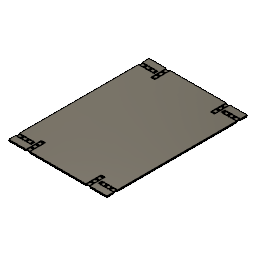
E-Reader Case v2 (Autodesk Fusion 360 design; units mm, degrees)
Autodesk Fusion 360 part; units mm, degrees
sketch "Sketch1" plane through (0, 0, 0) normal (0, 1, 0) x (1, 0, 0)
  line L0 (0, 0) -> (140, 0)
  line L1 (140, 0) -> (140, -200)
  line L2 (140, -200) -> (0, -200)
  line L3 (0, -200) -> (0, 0)
  dimension "d1" = 140
  dimension "d2" = 200
  constraint horizontal L0
  constraint vertical L1
  constraint horizontal L2
  constraint vertical L3
  constraint coincident L0.start L3.end
  measures "d1" distance of L0.start L0.end
  measures "d2" distance of L0.start L2.end
extrude "Extrude1" add sketch "Sketch1" along normal blind 2
sketch "Sketch2" plane through (0, 2, 0) normal (0, 1, 0) x (-1, 0, 0)
  line L0 (0, 200) -> (-140, 200)
  line L1 (-140, 200) -> (-140, 0)
  line L2 (-140, 0) -> (0, 0)
  line L3 (0, 0) -> (0, 200)
  line L4 (0, 0) -> (-30, 0)
  line L5 (-30, 0) -> (-30, 15)
  line L6 (-30, 15) -> (0, 15)
  line L7 (0, 15) -> (0, 0)
  line L8 (-140, 0) -> (-110, 0)
  line L9 (-110, 0) -> (-110, 15)
  line L10 (-110, 15) -> (-140, 15)
  line L11 (-140, 15) -> (-140, 0)
  line L12 (0, 200) -> (-30, 200)
  line L13 (-30, 200) -> (-30, 185)
  line L14 (-30, 185) -> (0, 185)
  line L15 (0, 185) -> (0, 200)
  line L16 (-140, 200) -> (-110, 200)
  line L17 (-110, 200) -> (-110, 185)
  line L18 (-110, 185) -> (-140, 185)
  line L19 (-140, 185) -> (-140, 200)
  line L20 (-110, 200) -> (-113, 200)
  line L21 (-140, 185) -> (-139, 185)
  line L22 (-110, 200) -> (-110, 199)
  line L23 (-120.831, 200) -> (-110, 200)
  line L24 (-110, 200) -> (-110, 199)
  line L25 (-30, 200) -> (-25, 200)
  line L26 (-25, 200) -> (-25, 199)
  line L27 (-25, 199) -> (-30, 199)
  line L28 (-30, 199) -> (-30, 200)
  line L29 (0, 185) -> (-1, 185)
  line L30 (-1, 185) -> (-1, 190)
  line L31 (-1, 190) -> (0, 190)
  line L32 (0, 190) -> (0, 185)
  line L33 (-140, 15) -> (-139, 15)
  line L34 (-139, 15) -> (-139, 10)
  line L35 (-139, 10) -> (-140, 10)
  line L36 (-140, 10) -> (-140, 15)
  line L37 (-110, 0) -> (-115, 0)
  line L38 (-115, 0) -> (-115, 1)
  line L39 (-115, 1) -> (-110, 1)
  line L40 (-110, 1) -> (-110, 0)
  line L41 (-30, 0) -> (-25, 0)
  line L42 (-25, 0) -> (-25, 1)
  line L43 (-25, 1) -> (-30, 1)
  line L44 (-30, 1) -> (-30, 0)
  line L45 (0, 15) -> (-1, 15)
  line L46 (-1, 15) -> (-1, 10)
  line L47 (-1, 10) -> (0, 10)
  line L48 (0, 10) -> (0, 15)
  line L49 (-140, 185) -> (-139, 185)
  line L50 (-139, 185) -> (-139, 190)
  line L51 (-139, 190) -> (-140, 190)
  line L52 (-140, 190) -> (-140, 185)
  line L53 (-110, 200) -> (-115, 200)
  line L54 (-115, 200) -> (-115, 199)
  line L55 (-115, 199) -> (-110, 199)
  line L56 (-110, 199) -> (-110, 200)
  dimension "d5" = 30
  dimension "d6" = 15
  dimension "d7" = 30
  dimension "d8" = 15
  dimension "d9" = 30
  dimension "d10" = 15
  dimension "d11" = 30
  dimension "d12" = 15
  dimension "d13" = 3
  dimension "d18" = 1
  dimension "d19" = 1
  dimension "d20" = 5
  dimension "d21" = 1
  dimension "d22" = 1
  dimension "d23" = 5
  dimension "d24" = 1
  dimension "d25" = 5
  dimension "d26" = 5
  dimension "d27" = 1
  dimension "d28" = 5
  dimension "d29" = 1
  dimension "d30" = 1
  dimension "d31" = 5
  dimension "d34" = 1
  dimension "d35" = 5
  dimension "d36" = 5
  dimension "d37" = 1
  constraint horizontal L4
  constraint vertical L5
  constraint horizontal L6
  constraint vertical L7
  constraint coincident L2.end L3.start
  constraint horizontal L8
  constraint vertical L9
  constraint horizontal L10
  constraint vertical L11
  constraint coincident L1.end L2.start
  constraint horizontal L12
  constraint vertical L13
  constraint horizontal L14
  constraint vertical L15
  constraint coincident L0.start L3.end
  constraint horizontal L16
  constraint vertical L17
  constraint horizontal L18
  constraint vertical L19
  constraint coincident L0.end L1.start
  constraint perpendicular L17 L20
  constraint horizontal L21
  constraint perpendicular L20 L22
  constraint horizontal L23
  constraint vertical L24
  constraint coincident L16 L23.start
  constraint horizontal L25
  constraint vertical L26
  constraint horizontal L27
  constraint vertical L28
  constraint horizontal L29
  constraint vertical L30
  constraint horizontal L31
  constraint vertical L32
  constraint horizontal L33
  constraint vertical L34
  constraint horizontal L35
  constraint vertical L36
  constraint horizontal L37
  constraint vertical L38
  constraint horizontal L39
  constraint vertical L40
  constraint horizontal L41
  constraint vertical L42
  constraint horizontal L43
  constraint vertical L44
  constraint horizontal L45
  constraint vertical L46
  constraint horizontal L47
  constraint vertical L48
  constraint horizontal L49
  constraint vertical L50
  constraint horizontal L51
  constraint vertical L52
  constraint horizontal L53
  constraint vertical L54
  constraint horizontal L55
  constraint vertical L56
  measures "d5" distance of L2.end L4.end
  measures "d6" distance of L2.end L6.end
  measures "d7" distance of L1.end L8.end
  measures "d8" distance of L1.end L10.end
  measures "d9" distance of L0.start L12.end
  measures "d10" distance of L0.start L14.end
  measures "d11" distance of L0.end L16.end
  measures "d12" distance of L0.end L18.end
  measures "d13" distance of L16.end L20.end
  measures "d18" distance of L18.end L21.end
  measures "d19" distance of L16.end L22.end
  measures "d20" distance of L12.end L25.end
  measures "d21" distance of L12.end L27.end
  measures "d22" distance of L14.end L29.end
  measures "d23" distance of L14.end L31.end
  measures "d24" distance of L10.end L33.end
  measures "d25" distance of L10.end L35.end
  measures "d26" distance of L8.end L37.end
  measures "d27" distance of L8.end L39.end
  measures "d28" distance of L4.end L41.end
  measures "d29" distance of L4.end L43.end
  measures "d30" distance of L6.end L45.end
  measures "d31" distance of L6.end L47.end
  measures "d34" distance of L18.end L21.end
  measures "d35" distance of L18.end L51.end
  measures "d36" distance of L16.end L53.end
  measures "d37" distance of L16.end L22.end
extrude "Extrude2" cut sketch "Sketch2" against normal blind 2 contours L0 L12 L13 L25 L26 L27 L28 | L3 L14 L15 L29 L30 L31 L32 | L0 L16 L17 L20 L22 L23 L24 L53 L54 L55 L56 | L3 L6 L7 L45 L46 L47 L48 | L1 L18 L19 L21 L49 L50 L51 L52 | L2 L4 L5 L41 L42 L43 L44 | L1 L10 L11 L33 L34 L35 L36 | L2 L8 L9 L37 L38 L39 L40
sketch "Sketch3" plane through (0, 2, 0) normal (0, 1, 0) x (-1, 0, 0)
  line L0 (-110, 1) -> (-110, 0)
  line L1 (-110, 0) -> (-30, 0)
  line L2 (-30, 0) -> (-30, 1)
  line L3 (-30, 1) -> (-25, 1)
  line L4 (-25, 0) -> (0, 0)
  line L5 (0, 0) -> (0, 10)
  line L6 (0, 10) -> (-1, 10)
  line L7 (-1, 10) -> (-1, 15)
  line L8 (-1, 15) -> (0, 15)
  line L9 (0, 15) -> (0, 185)
  line L10 (0, 185) -> (-1, 185)
  line L11 (-1, 185) -> (-1, 190)
  line L12 (-1, 190) -> (0, 190)
  line L13 (0, 190) -> (0, 200)
  line L14 (0, 200) -> (-25, 200)
  line L15 (-25, 200) -> (-25, 199)
  line L16 (-25, 199) -> (-30, 199)
  line L17 (-30, 199) -> (-30, 200)
  line L18 (-30, 200) -> (-110, 200)
  line L19 (-110, 200) -> (-110, 199)
  line L20 (-110, 199) -> (-115, 199)
  line L21 (-115, 199) -> (-115, 200)
  line L22 (-115, 200) -> (-140, 200)
  line L23 (-140, 200) -> (-140, 190)
  line L24 (-140, 190) -> (-139, 190)
  line L25 (-139, 190) -> (-139, 185)
  line L26 (-139, 185) -> (-140, 185)
  line L27 (-140, 185) -> (-140, 15)
  line L28 (-140, 15) -> (-139, 15)
  line L29 (-139, 15) -> (-139, 10)
  line L30 (-139, 10) -> (-140, 10)
  line L31 (-140, 10) -> (-140, 0)
  line L32 (-140, 0) -> (-115, 0)
  line L33 (-115, 1) -> (-110, 1)
  line L34 (-110, 199) -> (-115, 199)
  line L35 (-115, 199) -> (-115, 194)
  line L36 (-115, 194) -> (-110, 194)
  line L37 (-110, 194) -> (-110, 199)
  line L38 (-110, 194) -> (-115, 194)
  line L39 (-115, 194) -> (-115, 192)
  line L40 (-115, 192) -> (-110, 192)
  line L41 (-110, 192) -> (-110, 194)
  line L42 (-115, 192) -> (-110, 192)
  line L43 (-110, 192) -> (-110, 187)
  line L44 (-110, 187) -> (-115, 187)
  line L45 (-115, 187) -> (-115, 192)
  line L46 (-110, 187) -> (-115, 187)
  line L47 (-115, 187) -> (-115, 185)
  line L48 (-115, 185) -> (-110, 185)
  line L49 (-110, 185) -> (-110, 187)
  line L50 (-139, 185) -> (-134, 185)
  line L51 (-134, 185) -> (-134, 190)
  line L52 (-134, 190) -> (-139, 190)
  line L53 (-139, 190) -> (-139, 185)
  line L54 (-134, 190) -> (-132, 190)
  line L55 (-132, 190) -> (-132, 185)
  line L56 (-132, 185) -> (-134, 185)
  line L57 (-134, 185) -> (-134, 190)
  line L58 (-132, 185) -> (-127, 185)
  line L59 (-127, 185) -> (-127, 190)
  line L60 (-127, 190) -> (-132, 190)
  line L61 (-132, 190) -> (-132, 185)
  line L62 (-127, 190) -> (-125, 190)
  line L63 (-125, 190) -> (-125, 185)
  line L64 (-125, 185) -> (-127, 185)
  line L65 (-127, 185) -> (-127, 190)
  line L66 (-25, 199) -> (-30, 199)
  line L67 (-30, 199) -> (-30, 194)
  line L68 (-30, 194) -> (-25, 194)
  line L69 (-25, 194) -> (-25, 199)
  line L70 (-30, 194) -> (-25, 194)
  line L71 (-25, 194) -> (-25, 192)
  line L72 (-25, 192) -> (-30, 192)
  line L73 (-30, 192) -> (-30, 194)
  line L74 (-25, 192) -> (-30, 192)
  line L75 (-30, 192) -> (-30, 187)
  line L76 (-30, 187) -> (-25, 187)
  line L77 (-25, 187) -> (-25, 192)
  line L78 (-25, 187) -> (-30, 187)
  line L79 (-30, 187) -> (-30, 185)
  line L80 (-30, 185) -> (-25, 185)
  line L81 (-25, 185) -> (-25, 187)
  line L82 (-30, 185) -> (-25, 185)
  line L83 (-25, 185) -> (-25, 180)
  line L84 (-25, 180) -> (-30, 180)
  line L85 (-30, 180) -> (-30, 185)
  line L86 (-110, 185) -> (-115, 185)
  line L87 (-115, 185) -> (-115, 180)
  line L88 (-115, 180) -> (-110, 180)
  line L89 (-110, 180) -> (-110, 185)
  line L90 (-125, 185) -> (-120, 185)
  line L91 (-120, 185) -> (-120, 190)
  line L92 (-120, 190) -> (-125, 190)
  line L93 (-125, 190) -> (-125, 185)
  line L94 (-1, 185) -> (-6, 185)
  line L95 (-6, 185) -> (-6, 190)
  line L96 (-6, 190) -> (-1, 190)
  line L97 (-1, 190) -> (-1, 185)
  line L98 (-6, 190) -> (-8, 190)
  line L99 (-8, 190) -> (-8, 185)
  line L100 (-8, 185) -> (-6, 185)
  line L101 (-6, 185) -> (-6, 190)
  line L102 (-8, 185) -> (-13, 185)
  line L103 (-13, 185) -> (-13, 190)
  line L104 (-13, 190) -> (-8, 190)
  line L105 (-8, 190) -> (-8, 185)
  line L106 (-13, 190) -> (-15, 190)
  line L107 (-15, 190) -> (-15, 185)
  line L108 (-15, 185) -> (-13, 185)
  line L109 (-13, 185) -> (-13, 190)
  line L110 (-15, 185) -> (-20, 185)
  line L111 (-20, 185) -> (-20, 190)
  line L112 (-20, 190) -> (-15, 190)
  line L113 (-15, 190) -> (-15, 185)
  line L114 (-120, 15) -> (-125, 15)
  line L115 (-125, 10) -> (-120, 10)
  line L116 (-132, 15) -> (-132, 10)
  line L117 (-125, 15) -> (-125, 10)
  line L118 (-125, 10) -> (-127, 10)
  line L119 (-127, 10) -> (-127, 15)
  line L120 (-134, 15) -> (-132, 15)
  line L121 (-139, 10) -> (-134, 10)
  line L122 (-127, 15) -> (-132, 15)
  line L123 (-127, 10) -> (-127, 15)
  line L124 (-134, 10) -> (-134, 15)
  line L125 (-127, 15) -> (-125, 15)
  line L126 (-125, 15) -> (-125, 10)
  line L127 (-134, 15) -> (-139, 15)
  line L128 (-132, 10) -> (-134, 10)
  line L129 (-132, 10) -> (-127, 10)
  line L130 (-139, 15) -> (-139, 10)
  line L131 (-134, 10) -> (-134, 15)
  line L132 (-132, 15) -> (-132, 10)
  line L133 (-139, 15) -> (-139, 10)
  line L134 (-1, 15) -> (-6, 15)
  line L135 (-6, 10) -> (-1, 10)
  line L136 (-13, 15) -> (-13, 10)
  line L137 (-6, 15) -> (-6, 10)
  line L138 (-6, 10) -> (-8, 10)
  line L139 (-8, 10) -> (-8, 15)
  line L140 (-15, 15) -> (-13, 15)
  line L141 (-20, 10) -> (-15, 10)
  line L142 (-8, 15) -> (-13, 15)
  line L143 (-8, 10) -> (-8, 15)
  line L144 (-15, 10) -> (-15, 15)
  line L145 (-8, 15) -> (-6, 15)
  line L146 (-6, 15) -> (-6, 10)
  line L147 (-1, 12) -> (-1, 10)
  line L148 (-15, 15) -> (-20, 15)
  line L149 (-13, 10) -> (-15, 10)
  line L150 (-13, 10) -> (-8, 10)
  line L151 (-15, 10) -> (-15, 15)
  line L152 (-13, 15) -> (-13, 10)
  line L153 (-1, 10) -> (-1, 15)
  line L154 (-120, 190) -> (-118, 190)
  line L155 (-118, 190) -> (-118, 185)
  line L156 (-118, 185) -> (-120, 185)
  line L157 (-120, 185) -> (-120, 190)
  line L158 (-110, 180) -> (-115, 180)
  line L159 (-115, 180) -> (-115, 178)
  line L160 (-115, 178) -> (-110, 178)
  line L161 (-110, 178) -> (-110, 180)
  line L162 (-20, 185) -> (-22, 185)
  line L163 (-22, 185) -> (-22, 190)
  line L164 (-22, 190) -> (-20, 190)
  line L165 (-20, 190) -> (-20, 185)
  line L166 (-25, 180) -> (-30, 180)
  line L167 (-30, 180) -> (-30, 178)
  line L168 (-30, 178) -> (-25, 178)
  line L169 (-25, 178) -> (-25, 180)
  line L170 (-20, 15) -> (-20, 10)
  line L171 (-20, 15) -> (-22, 15)
  line L172 (-22, 15) -> (-22, 10)
  line L173 (-22, 10) -> (-20, 10)
  line L174 (-20, 10) -> (-20, 15)
  line L175 (-120, 15) -> (-118, 15)
  line L176 (-118, 15) -> (-118, 10)
  line L177 (-118, 10) -> (-120, 10)
  line L178 (-120, 10) -> (-120, 15)
  line L179 (-115, 8) -> (-115, 13)
  line L180 (-110, 13) -> (-110, 15)
  line L181 (-115, 13) -> (-110, 13)
  line L182 (-110, 20) -> (-115, 20)
  line L183 (-115, 6) -> (-115, 1)
  line L184 (-110, 6) -> (-115, 6)
  line L185 (-110, 8) -> (-115, 8)
  line L186 (-115, 15) -> (-115, 13)
  line L187 (-110, 8) -> (-115, 8)
  line L188 (-110, 20) -> (-115, 20)
  line L189 (-110, 15) -> (-110, 20)
  line L190 (-115, 13) -> (-110, 13)
  line L191 (-110, 13) -> (-110, 8)
  line L192 (-110, 1) -> (-115, 1)
  line L193 (-115, 8) -> (-115, 6)
  line L194 (-115, 20) -> (-115, 15)
  line L195 (-115, 1) -> (-110, 1)
  line L196 (-115, 6) -> (-110, 6)
  line L197 (-115, 15) -> (-110, 15)
  line L198 (-110, 6) -> (-110, 8)
  line L199 (-110, 15) -> (-115, 15)
  line L200 (-110, 1) -> (-110, 6)
  line L201 (-30, 8) -> (-30, 13)
  line L202 (-25, 13) -> (-25, 15)
  line L203 (-30, 13) -> (-25, 13)
  line L204 (-25, 20) -> (-30, 20)
  line L205 (-30, 6) -> (-30, 1)
  line L206 (-25, 6) -> (-30, 6)
  line L207 (-25, 8) -> (-30, 8)
  line L208 (-30, 15) -> (-30, 13)
  line L209 (-25, 8) -> (-30, 8)
  line L210 (-25, 20) -> (-30, 20)
  line L211 (-25, 15) -> (-25, 20)
  line L212 (-30, 13) -> (-25, 13)
  line L213 (-25, 13) -> (-25, 8)
  line L214 (-25, 1) -> (-30, 1)
  line L215 (-30, 8) -> (-30, 6)
  line L216 (-30, 20) -> (-30, 15)
  line L217 (-30, 1) -> (-25, 1)
  line L218 (-30, 6) -> (-25, 6)
  line L219 (-30, 15) -> (-25, 15)
  line L220 (-25, 6) -> (-25, 8)
  line L221 (-25, 15) -> (-30, 15)
  line L222 (-25, 1) -> (-25, 6)
  line L223 (-25, 20) -> (-30, 20)
  line L224 (-30, 20) -> (-30, 22)
  line L225 (-30, 22) -> (-25, 22)
  line L226 (-25, 22) -> (-25, 20)
  line L227 (-110, 20) -> (-115, 20)
  line L228 (-115, 20) -> (-115, 22)
  line L229 (-115, 22) -> (-110, 22)
  line L230 (-110, 22) -> (-110, 20)
  point P0 (-1, 10)
  point P1 (-1, 12)
  dimension "d38" = 5
  dimension "d39" = 5
  dimension "d40" = 5
  dimension "d41" = 2
  dimension "d42" = 5
  dimension "d43" = 5
  dimension "d44" = 5
  dimension "d45" = 2
  dimension "d46" = 5
  dimension "d47" = 5
  dimension "d48" = 2
  dimension "d49" = 5
  dimension "d50" = 5
  dimension "d51" = 5
  dimension "d52" = 2
  dimension "d53" = 5
  dimension "d54" = 5
  dimension "d55" = 5
  dimension "d56" = 5
  dimension "d57" = 2
  dimension "d58" = 5
  dimension "d59" = 5
  dimension "d60" = 5
  dimension "d61" = 2
  dimension "d62" = 5
  dimension "d63" = 5
  dimension "d64" = 5
  dimension "d65" = 5
  dimension "d66" = 5
  dimension "d67" = 5
  dimension "d68" = 5
  dimension "d69" = 5
  dimension "d70" = 2
  dimension "d71" = 5
  dimension "d72" = 5
  dimension "d73" = 5
  dimension "d74" = 2
  dimension "d75" = 5
  dimension "d76" = 5
  dimension "d77" = 5
  dimension "d78" = 5
  dimension "d79" = 5
  dimension "d80" = 2
  dimension "d81" = 5
  dimension "d82" = 5
  dimension "d83" = 5
  dimension "d84" = 2
  dimension "d85" = 5
  dimension "d86" = 5
  dimension "d87" = 5
  dimension "d88" = 5
  dimension "d90" = 2
  dimension "d91" = 5
  dimension "d92" = 5
  dimension "d93" = 5
  dimension "d94" = 2
  dimension "d95" = 5
  dimension "d96" = 5
  dimension "d97" = 5
  dimension "d126" = 2
  dimension "d127" = 5
  dimension "d128" = 2
  dimension "d129" = 2
  dimension "d130" = 5
  dimension "d131" = 2
  dimension "d132" = 2
  dimension "d133" = 2
  dimension "d134" = 5
  dimension "d135" = 5
  dimension "d136" = 5
  dimension "d137" = 2
  dimension "d138" = 5
  dimension "d139" = 5
  dimension "d140" = 5
  dimension "d141" = 2
  dimension "d142" = 5
  dimension "d143" = 5
  dimension "d144" = 5
  dimension "d145" = 5
  dimension "d146" = 5
  dimension "d147" = 5
  dimension "d148" = 2
  dimension "d149" = 5
  dimension "d150" = 5
  dimension "d151" = 5
  dimension "d152" = 2
  dimension "d153" = 5
  dimension "d154" = 5
  dimension "d155" = 5
  dimension "d156" = 2
  dimension "d157" = 2
  constraint horizontal L34
  constraint vertical L35
  constraint horizontal L36
  constraint vertical L37
  constraint coincident L19.end L20.start
  constraint horizontal L38
  constraint vertical L39
  constraint horizontal L40
  constraint vertical L41
  constraint horizontal L42
  constraint vertical L43
  constraint horizontal L44
  constraint vertical L45
  constraint horizontal L46
  constraint vertical L47
  constraint horizontal L48
  constraint vertical L49
  constraint horizontal L50
  constraint vertical L51
  constraint horizontal L52
  constraint vertical L53
  constraint coincident L25.end L26.start
  constraint horizontal L54
  constraint vertical L55
  constraint horizontal L56
  constraint vertical L57
  constraint horizontal L58
  constraint vertical L59
  constraint horizontal L60
  constraint vertical L61
  constraint horizontal L62
  constraint vertical L63
  constraint horizontal L64
  constraint vertical L65
  constraint horizontal L66
  constraint vertical L67
  constraint horizontal L68
  constraint vertical L69
  constraint coincident L15.end L16.start
  constraint horizontal L70
  constraint vertical L71
  constraint horizontal L72
  constraint vertical L73
  constraint horizontal L74
  constraint vertical L75
  constraint horizontal L76
  constraint vertical L77
  constraint horizontal L78
  constraint vertical L79
  constraint horizontal L80
  constraint vertical L81
  constraint horizontal L82
  constraint vertical L83
  constraint horizontal L84
  constraint vertical L85
  constraint horizontal L86
  constraint vertical L87
  constraint horizontal L88
  constraint vertical L89
  constraint horizontal L90
  constraint vertical L91
  constraint horizontal L92
  constraint vertical L93
  constraint horizontal L94
  constraint vertical L95
  constraint horizontal L96
  constraint vertical L97
  constraint coincident L10.end L11.start
  constraint horizontal L98
  constraint vertical L99
  constraint horizontal L100
  constraint vertical L101
  constraint horizontal L102
  constraint vertical L103
  constraint horizontal L104
  constraint vertical L105
  constraint horizontal L106
  constraint vertical L107
  constraint horizontal L108
  constraint vertical L109
  constraint horizontal L110
  constraint vertical L111
  constraint horizontal L112
  constraint vertical L113
  constraint horizontal L121
  constraint vertical L124
  constraint horizontal L127
  constraint vertical L130
  constraint coincident L29.end L30.start
  constraint horizontal L120
  constraint vertical L132
  constraint horizontal L128
  constraint vertical L131
  constraint horizontal L129
  constraint vertical L123
  constraint horizontal L122
  constraint vertical L116
  constraint horizontal L125
  constraint vertical L117
  constraint horizontal L118
  constraint vertical L119
  constraint horizontal L115
  constraint horizontal L114
  constraint vertical L126
  constraint vertical L147
  constraint horizontal L141
  constraint vertical L144
  constraint horizontal L148
  constraint horizontal L140
  constraint vertical L152
  constraint horizontal L149
  constraint vertical L151
  constraint horizontal L150
  constraint vertical L143
  constraint horizontal L142
  constraint vertical L136
  constraint horizontal L145
  constraint vertical L137
  constraint horizontal L138
  constraint vertical L139
  constraint horizontal L135
  constraint vertical L153
  constraint horizontal L134
  constraint vertical L146
  constraint horizontal L154
  constraint vertical L155
  constraint horizontal L156
  constraint vertical L157
  constraint horizontal L158
  constraint vertical L159
  constraint horizontal L160
  constraint vertical L161
  constraint horizontal L162
  constraint vertical L163
  constraint horizontal L164
  constraint vertical L165
  constraint horizontal L166
  constraint vertical L167
  constraint horizontal L168
  constraint vertical L169
  constraint perpendicular L141 L170
  constraint horizontal L171
  constraint vertical L172
  constraint horizontal L173
  constraint vertical L174
  constraint horizontal L175
  constraint vertical L176
  constraint horizontal L177
  constraint vertical L178
  constraint horizontal L188
  constraint vertical L194
  constraint horizontal L197
  constraint vertical L189
  constraint coincident L182.start L188.start
  constraint horizontal L199
  constraint vertical L186
  constraint horizontal L181
  constraint vertical L180
  constraint horizontal L190
  constraint vertical L191
  constraint horizontal L185
  constraint vertical L179
  constraint horizontal L187
  constraint vertical L193
  constraint horizontal L196
  constraint vertical L198
  constraint horizontal L184
  constraint vertical L183
  constraint horizontal L195
  constraint vertical L200
  constraint horizontal L192
  constraint horizontal L210
  constraint vertical L216
  constraint horizontal L219
  constraint vertical L211
  constraint coincident L204.start L210.start
  constraint horizontal L221
  constraint vertical L208
  constraint horizontal L203
  constraint vertical L202
  constraint horizontal L212
  constraint vertical L213
  constraint horizontal L207
  constraint vertical L201
  constraint horizontal L209
  constraint vertical L215
  constraint horizontal L218
  constraint vertical L220
  constraint horizontal L206
  constraint vertical L205
  constraint horizontal L217
  constraint vertical L222
  constraint horizontal L214
  constraint horizontal L223
  constraint vertical L224
  constraint horizontal L225
  constraint vertical L226
  constraint horizontal L227
  constraint vertical L228
  constraint horizontal L229
  constraint vertical L230
  measures "d38" distance of L19.end L20.end
  measures "d39" distance of L19.end L36.end
  measures "d40" distance of L36.end L35.end
  measures "d41" distance of L36.end L40.end
  measures "d42" distance of L39.end L40.end
  measures "d43" distance of L39.end L44.end
  measures "d44" distance of L43.end L44.end
  measures "d45" distance of L43.end L48.end
  measures "d46" distance of L25.end L50.end
  measures "d47" distance of L25.end L24.end
  measures "d48" distance of L51.end L54.end
  measures "d49" distance of L51.end L50.end
  measures "d50" distance of L55.end L58.end
  measures "d51" distance of L55.end L54.end
  measures "d52" distance of L59.end L62.end
  measures "d53" distance of L59.end L58.end
  measures "d54" distance of L15.end L16.end
  measures "d55" distance of L15.end L68.end
  measures "d56" distance of L67.end L68.end
  measures "d57" distance of L67.end L72.end
  measures "d58" distance of L71.end L72.end
  measures "d59" distance of L71.end L76.end
  measures "d60" distance of L76.end L75.end
  measures "d61" distance of L76.end L80.end
  measures "d62" distance of L79.end L80.end
  measures "d63" distance of L79.end L84.end
  measures "d64" distance of L48.end L47.end
  measures "d65" distance of L48.end L88.end
  measures "d66" distance of L63.end L90.end
  measures "d67" distance of L63.end L62.end
  measures "d68" distance of L10.end L94.end
  measures "d69" distance of L10.end L11.end
  measures "d70" distance of L95.end L98.end
  measures "d71" distance of L95.end L94.end
  measures "d72" distance of L99.end L102.end
  measures "d73" distance of L99.end L98.end
  measures "d74" distance of L103.end L106.end
  measures "d75" distance of L103.end L102.end
  measures "d76" distance of L107.end L110.end
  measures "d77" distance of L107.end L106.end
  measures "d78" distance of L29.end L121.end
  measures "d79" distance of L29.end L28.end
  measures "d80" distance of L116.start L120.start
  measures "d81" distance of L120.start L121.end
  measures "d82" distance of L118.end L116.end
  measures "d83" distance of L116.end L116.start
  measures "d84" distance of L114.end L119.end
  measures "d85" distance of L118.end L119.end
  measures "d86" distance of L115.start L115.end
  measures "d87" distance of L115.start L114.end
  measures "d88" distance of L141.start L141.end
  measures "d90" distance of L136.start L140.start
  measures "d91" distance of L140.start L141.end
  measures "d92" distance of L138.end L136.end
  measures "d93" distance of L136.end L136.start
  measures "d94" distance of L134.end L139.end
  measures "d95" distance of L138.end L139.end
  measures "d96" distance of L135.start P0
  measures "d97" distance of L135.start L134.end
  measures "d126" distance of L91.end L154.end
  measures "d127" distance of L88.end L87.end
  measures "d128" distance of L88.end L160.end
  measures "d129" distance of L110.end L162.end
  measures "d130" distance of L110.end L111.end
  measures "d131" distance of L83.end L168.end
  measures "d132" distance of L148.end L171.end
  measures "d133" distance of L114.start L175.end
  measures "d134" distance of L182.end L182.start
  measures "d135" distance of L180.end L182.start
  measures "d136" distance of L186.start L180.end
  measures "d137" distance of L180.end L180.start
  measures "d138" distance of L179.end L180.start
  measures "d139" distance of L179.start L179.end
  measures "d140" distance of L179.start L185.start
  measures "d141" distance of L185.start L184.start
  measures "d142" distance of L183.start L184.start
  measures "d143" distance of L184.start L0.start
  measures "d144" distance of L0.start L33.start
  measures "d145" distance of L204.end L204.start
  measures "d146" distance of L202.end L204.start
  measures "d147" distance of L208.start L202.end
  measures "d148" distance of L202.end L202.start
  measures "d149" distance of L201.end L202.start
  measures "d150" distance of L201.start L201.end
  measures "d151" distance of L201.start L207.start
  measures "d152" distance of L207.start L206.start
  measures "d153" distance of L205.start L206.start
  measures "d154" distance of L206.start L3.end
  measures "d155" distance of L3.end L2.end
  measures "d156" distance of L204.start L225.end
  measures "d157" distance of L182.start L229.end
extrude "Extrude3" cut sketch "Sketch3" against normal blind 2 contours L206 L207 L209 L215 L218 L220 | L202 L203 L208 L212 L219 L221 | L204 L210 L223 L224 L225 L226 | L137 L138 L139 L143 L145 L146 | L136 L140 L144 L149 L151 L152 | L170 L171 L172 L173 L174 | L95 L98 L99 L100 L101 L105 | L103 L106 L107 L108 L109 L113 | L111 L162 L163 L164 L165 | L68 L70 L71 L72 L73 L74 | L76 L78 L79 L80 L81 L82 | L84 L166 L167 L168 L169 | L36 L38 L39 L40 L41 L42 | L44 L46 L47 L48 L49 L86 | L88 L158 L159 L160 L161 | L51 L54 L55 L56 L57 L61 | L59 L62 L63 L64 L65 L93 | L91 L154 L155 L156 L157 | L116 L120 L124 L128 L131 L132 | L117 L118 L119 L123 L125 L126 | L175 L176 L177 L178 | L184 L185 L187 L193 L196 L198 | L180 L181 L186 L190 L197 L199 | L182 L188 L227 L228 L229 L230
extrude "Extrude4" cut sketch "Sketch3" against normal blind 0.5 contours L3 L205 L206 L214 L217 L218 L222 | L201 L203 L207 L209 L212 L213 | L204 L210 L211 L216 L219 L221 L223 | L7 L134 L135 L137 L146 L147 L153 | L136 L139 L142 L143 L150 L152 | L141 L144 L148 L151 L170 L174 | L11 L94 L95 L96 L97 L101 | L99 L102 L103 L104 L105 L109 | L107 L110 L111 L112 L113 L165 | L16 L66 L67 L68 L69 L70 | L72 L74 L75 L76 L77 L78 | L80 L82 L83 L84 L85 L166 | L20 L34 L35 L36 L37 L38 | L40 L42 L43 L44 L45 L46 | L48 L86 L87 L88 L89 L158 | L25 L50 L51 L52 L53 L57 | L55 L58 L59 L60 L61 L65 | L63 L90 L91 L92 L93 L157 | L29 L121 L124 L127 L130 L131 L133 | L116 L119 L122 L123 L129 L132 | L114 L115 L117 L126 L178 | L33 L183 L184 L192 L195 L196 L200 | L179 L181 L185 L187 L190 L191 | L182 L188 L189 L194 L197 L199 L227
extrude "Extrude5" cut sketch "Sketch3" along normal blind -2 and the other way blind 1.5 contours L3 L205 L206 L214 L217 L218 L222 | L201 L203 L207 L209 L212 L213 | L204 L210 L211 L216 L219 L221 L223 | L7 L134 L135 L137 L146 L147 L153 | L136 L139 L142 L143 L150 L152 | L141 L144 L148 L151 L170 L174 | L11 L94 L95 L96 L97 L101 | L99 L102 L103 L104 L105 L109 | L107 L110 L111 L112 L113 L165 | L16 L66 L67 L68 L69 L70 | L72 L74 L75 L76 L77 L78 | L80 L82 L83 L84 L85 L166 | L20 L34 L35 L36 L37 L38 | L40 L42 L43 L44 L45 L46 | L48 L86 L87 L88 L89 L158 | L25 L50 L51 L52 L53 L57 | L55 L58 L59 L60 L61 L65 | L63 L90 L91 L92 L93 L157 | L29 L121 L124 L127 L130 L131 L133 | L116 L119 L122 L123 L129 L132 | L114 L115 L117 L126 L178 | L33 L183 L184 L192 L195 L196 L200 | L179 L181 L185 L187 L190 L191 | L182 L188 L189 L194 L197 L199 L227
